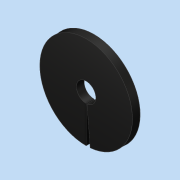
# Autodesk Inventor part: encoderDisc
Saved by Autodesk Inventor 2017 (Build 210142000, 142)
## iProperties
Created: 2016-12-12
Part Number: encoderDisc
Material: ABS Plastic
Document SubType Name: Modeling
Designer: techn
Density: 1.06 g/cm^3
Appearance: Glossy - Black
Author: techn
Autodesk Inventor part; units mm, degrees
ref_plane "YZ Plane" through (0, 0, 0) normal (1, 0, 0) x (0, 1, 0)
ref_plane "XZ Plane" through (0, 0, 0) normal (0, 1, 0) x (-1, 0, 0)
ref_plane "XY Plane" through (0, 0, 0) normal (0, 0, 1) x (1, 0, 0)
sketch "Sketch1" plane through (0, 0, 0) normal (0, 0, 1) x (1, 0, 0)
  circle A0 centre (0, 0) radius 9.525
  line L0 (0, 0) -> (0, -9.525)
  line L1 (0, 0) -> (0.8302, -9.4888)
  line L2 (0, 0) -> (9.525, 0) construction
  dimension "d0" = 19.05
  dimension "d1" = 85
  constraints: 6 end point, 2 point on circle, 1 centre point, 1 coincident, 1 equal length, 1 horizontal, 1 vertical
  measures "d0" diameter of A0
  measures "d1" angle of L1 L2
extrude "Extrusion1" add sketch "Sketch1" along normal blind 1.5875 contours A0 L1 L0 picked at (-0.7794, -6.2528)
sketch "Sketch2" plane through (0, 0, 1.5875) normal (0, 0, 1) x (1, 0, 0)
  circle A0 centre (0, 0) radius 2
  dimension "d4" = 4
  constraints: 1 centre point, 1 coincident
  measures "d4" diameter of A0
extrude "Extrusion2" cut sketch "Sketch2" against normal blind 1.5875
body "Solid1"
